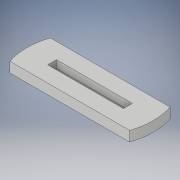
# Autodesk Inventor part: planetstand
Saved by Autodesk Inventor 2018 (Build 220112000, 112)
## iProperties
Created: 2017-12-11
Part Number: planetstand
Material: Generic
Document SubType Name: Modeling
Designer: lewisw19
Density: 1 g/cm^3
Appearance: Default
Author: lewisw19
Autodesk Inventor part; units mm, degrees
ref_plane "YZ Plane" through (0, 0, 0) normal (1, 0, 0) x (0, 1, 0)
ref_plane "XZ Plane" through (0, 0, 0) normal (0, 1, 0) x (-1, 0, 0)
ref_plane "XY Plane" through (0, 0, 0) normal (0, 0, 1) x (1, 0, 0)
sketch "Sketch1" plane through (0, 0, 0) normal (0, 1, 0) x (-1, 0, 0)
  circle A0 centre (0, 0) radius 25
  dimension "d2" = 50
  constraints: 1 centre point, 1 coincident
  measures "d2" diameter of A0
extrude "Extrusion1" add sketch "Sketch1" along normal blind 10
sketch "Sketch2" plane through (0, 10, 0) normal (0, 1, 0) x (1, 0, 0)
  line L0 (-15, -1.75) -> (15, -1.75)
  line L1 (15, -1.75) -> (15, 1.75)
  line L2 (15, 1.75) -> (-15, 1.75)
  line L3 (-15, 1.75) -> (-15, -1.75)
  circle A0 centre (0, 0) radius 25 projected
  point P0 (-25, 0)
  point P1 (0, 25)
  dimension "d5" = 30
  dimension "d6" = 3.5
  dimension "d7" = 23.25
  dimension "d8" = 10
  constraints: 8 end point, 2 parallel, 2 point on circle, 1 horizontal, 1 perpendicular
  measures "d5" distance of L2.end L1.end
  measures "d6" distance of L1.end L0.end
  measures "d7" distance from line of L2 A0.end
  measures "d8" distance from line of L3 A0.start
extrude "Extrusion2" cut sketch "Sketch2" against normal blind 3 contours L3 L2 L1 L0
sketch "Sketch3" plane through (0, 10, 0) normal (0, 1, 0) x (1, 0, 0)
  line L0 (-38.0663, 8) -> (91.0616, 8)
  line L1 (-15, 1.75) -> (15, 1.75) projected
  arc A0 (91.0616, 8) -> (-38.0663, 8) centre (26.4976, -23.1626) ccw
  circle A1 centre (0, 0) radius 25 construction
  line L2 (-25, 0) -> (81.9095, 0) construction
  line L3 (-38.0663, -8) -> (91.0616, -8)
  arc A2 (-38.0663, -8) -> (91.0616, -8) centre (26.4976, 23.1626) ccw
  point P0 (24.7878, -3.25)
  dimension "d11" = 6.25
  constraints: 6 end point, 5 point on circle, 3 symmetric about line, 2 centre point, 2 horizontal, 2 other
extrude "Extrusion3" cut sketch "Sketch3" against normal blind 10
sketch "Sketch4" plane through (0, 0, 0) normal (0, -1, 0) x (1, 0, 0)
  line L0 (-23.6854, -8) -> (23.6854, -8) projected
  arc A0 (23.6854, -8) -> (23.6854, 8) centre (0, 0) ccw projected
  line L1 (23.6854, 8) -> (-23.6854, 8) projected
  arc A1 (-23.6854, 8) -> (-23.6854, -8) centre (0, 0) ccw projected
extrude "Extrusion4" cut sketch "Sketch4" against normal blind 6
body "Solid1"
